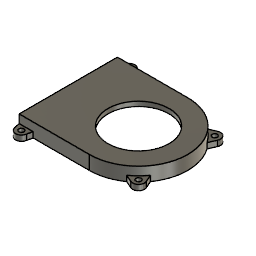
Rotor Housing v1 (Autodesk Fusion 360 design; units mm, degrees)
part number: 2026-05-21-21-26-19-566
Autodesk Fusion 360 part; units mm, degrees
sketch "Sketch1" plane through (0, 0, 0) normal (0, 0, 1) x (1, 0, 0)
  line L0 (0, 26.67) -> (-38.1, 26.67)
  line L1 (0, -26.67) -> (-38.1, -26.67)
  line L2 (-38.1, 24.257) -> (0, 24.257)
  line L3 (-38.1, -24.257) -> (0, -24.257)
  line L4 (-38.1, 26.67) -> (-38.1, 24.257)
  line L5 (-38.1, -24.257) -> (-38.1, -26.67)
  arc A0 (0, -26.67) -> (0, 26.67) centre (0, 0) ccw
  arc A1 (0, -24.257) -> (0, 24.257) centre (0, 0) ccw
  dimension "d1" = 53.34
  dimension "d2" = 48.514
  dimension "d3" = 38.1
  dimension "d4" = 38.1
  constraint coincident A0.centre A1.centre
  constraint horizontal L0
  constraint horizontal L1
  constraint tangent L0 A0
  constraint tangent L1 A0
  constraint horizontal L2
  constraint parallel L1 L3
  constraint tangent L2 A1
  constraint tangent L3 A1
  constraint vertical L4
  constraint perpendicular L1 L5
  constraint coincident L0.end L4.start
  constraint coincident L2.start L4.end
  constraint coincident L3.start L5.start
  constraint coincident L1.end L5.end
  measures "d1" diameter of A0
  measures "d2" diameter of A1
  measures "d3" distance of L0.start L0.end
  measures "d4" distance of L1.start L1.end
extrude "Extrude1" add sketch "Sketch1" along normal blind 5
sketch "Sketch2" plane through (0, 0, 5) normal (0, 0, 1) x (-1, 0, 0)
  line L0 (38.1, 24.257) -> (38.1, 26.67)
  line L1 (38.1, 26.67) -> (0, 26.67)
  arc A0 (0, 26.67) -> (0, -26.67) centre (0, 0) ccw
  line L2 (0, -26.67) -> (38.1, -26.67)
  line L3 (38.1, -26.67) -> (38.1, -24.257)
  line L4 (38.1, -24.257) -> (0, -24.257)
  arc A1 (0, 24.257) -> (0, -24.257) centre (0, 0) ccw
  line L5 (0, 24.257) -> (38.1, 24.257)
  line L6 (38.1, -26.67) -> (38.1, 26.67)
  constraint coincident L2.end L3.start
  constraint coincident L0.end L1.start
extrude "Extrude2" add sketch "Sketch2" along normal blind 2.54
sketch "Sketch3" plane through (0, 0, 7.54) normal (0, 0, 1) x (-1, 0, 0)
  line L0 (38.1, -26.67) -> (38.1, 26.67)
  line L1 (38.1, 26.67) -> (0, 26.67)
  arc A0 (0, 26.67) -> (0, -26.67) centre (0, 0) ccw
  line L2 (0, -26.67) -> (38.1, -26.67)
  circle A1 centre (0, 0) radius 16.51
  dimension "d9" = 33.02
  constraint concentric A0 A1
  measures "d9" diameter of A1
extrude "Extrude3" cut sketch "Sketch3" against normal through all contours A1
sketch "Sketch4" plane through (0, 0, 5) normal (0, 0, -1) x (1, 0, 0)
  circle A0 centre (0, 0) radius 16.51
  line L0 (0, 24.257) -> (-38.1, 24.257)
  line L1 (-38.1, 24.257) -> (-38.1, -24.257)
  line L2 (-38.1, -24.257) -> (0, -24.257)
  arc A1 (0, -24.257) -> (0, 24.257) centre (0, 0) ccw
  line L3 (-38.1, 19.257) -> (-35.56, 19.257)
  line L4 (-35.56, 19.257) -> (-35.56, -19.257)
  line L5 (-35.56, -19.257) -> (-38.1, -19.257)
  line L6 (-38.1, -19.257) -> (-38.1, 19.257)
  dimension "d11" = 5
  dimension "d12" = 5
  constraint horizontal L3
  constraint vertical L4
  constraint horizontal L5
  constraint vertical L6
  constraint coincident L1 L3.start
  measures "d11" distance of L0 L3
  measures "d12" distance of L2 L5
extrude "Extrude4" add sketch "Sketch4" along normal blind 5 contours L1 L3 L4 L5 L6
sketch "Sketch5" plane through (0, 0, 0) normal (0, 0, 1) x (1, 0, 0)
  line L0 (0, 0) -> (30.48, 30.48) construction
  line L1 (0, 0) -> (43.1052, 0) construction
  line L2 (0, 0) -> (33.4313, -33.4313) construction
  line L3 (0, 0) -> (47.279, 0) construction
  circle A0 centre (20.6546, 20.6546) radius 1.4
  circle A1 centre (20.6546, -20.6546) radius 1.4
  circle A2 centre (20.6546, 20.6546) radius 3.175
  line L4 (19.3121, 23.5318) -> (15.3534, 21.8074)
  line L5 (23.5318, 19.3121) -> (21.8074, 15.3534)
  arc A3 (0, -26.67) -> (0, 26.67) centre (0, 0) ccw
  dimension "d15" = 45
  dimension "d16" = 45
  dimension "d17" = 2.8
  dimension "d18" = 2.8
  dimension "d19" = 29.21
  dimension "d20" = 29.21
  dimension "d21" = 6.35
  dimension "d22" = 4.318
  constraint horizontal L1
  constraint coincident L0.start L1.start
  constraint horizontal L3
  constraint coincident L0 A0.centre
  constraint coincident L2 A1.centre
  constraint concentric A0 A2
  constraint coincident A2 L4.start
  constraint coincident A2 L5.start
  constraint coincident L4.end A3
  constraint coincident L5.end A3
  constraint symmetric L0 L4 L5
  measures "d15" angle of L0 L1
  measures "d16" angle of L2 L3
  measures "d17" diameter of A1
  measures "d18" diameter of A0
  measures "d19" distance of L0.start A1.centre
  measures "d20" distance of L0.start A0.centre
  measures "d21" diameter of A2
  measures "d22" distance of L4.start L4.end
extrude "Extrude5" add sketch "Sketch5" along normal blind 3 contours A2 A3 | A2 L4 A3 | A2 L5 A3 picked at (18.4077, 19.9432)
mirror "Mirror1" about plane through (0, 0, 0) normal (0, 1, 0) of "Extrude5"
sketch "Sketch6" plane through (0, 0, 0) normal (0, 0, 1) x (1, 0, 0)
  circle A0 centre (-34.29, -29.21) radius 1.4
  line L0 (-38.1, 26.67) -> (-38.1, -26.67)
  line L1 (-38.1, -26.67) -> (0, -26.67)
  circle A1 centre (-34.29, -29.21) radius 3.175
  line L2 (-37.444, -29.5746) -> (-38.1, -26.67)
  line L3 (-31.136, -29.5746) -> (-30.48, -26.67)
  dimension "d27" = 2.8
  dimension "d28" = 3.81
  dimension "d29" = 2.54
  dimension "d30" = 6.35
  constraint concentric A0 A1
  constraint coincident A1 L2.start
  constraint coincident L0.end L1.start
  constraint coincident A1 L3.start
  constraint coincident L1 L3.end
  measures "d27" diameter of A0
  measures "d28" distance of A0.centre L0
  measures "d29" distance of A0.centre L1
  measures "d30" diameter of A1
extrude "Extrude6" add sketch "Sketch6" along normal blind 3 contours L1 A1 L2 | L1 A1 | L1 A1 L3 picked at (-34.3249, -27.0513)
mirror "Mirror2" about plane through (0, 0, 0) normal (0, 1, 0) of "Extrude6"
sketch "Sketch7" plane through (0, 0, 0) normal (0, 0, 1) x (1, 0, 0)
  line L0 (38.1, -38.1) -> (-38.1, -38.1) construction
  line L1 (-38.1, -38.1) -> (-38.1, 38.1) construction
  line L2 (-38.1, 38.1) -> (38.1, 38.1) construction
  line L3 (38.1, 38.1) -> (38.1, -38.1) construction
  line L4 (38.1, -38.1) -> (-38.1, 38.1) construction
  line L5 (-38.1, -38.1) -> (38.1, 38.1) construction
  dimension "d35" = 76.2
  dimension "d36" = 76.2
  constraint horizontal L0
  constraint perpendicular L0 L1
  constraint parallel L0 L2
  constraint parallel L1 L3
  constraint coincident L4 origin
  constraint coincident L5 origin
  measures "d35" distance of L1.end L2.end
  measures "d36" distance of L0.end L1.end
